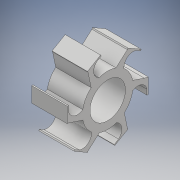
# Autodesk Inventor part: mtv_gear6_1-15
Saved by Autodesk Inventor 2018 (Build 220112000, 112)
## iProperties
Created: 2019-01-16
Part Number: mtv_gear6_1-15
Material: Generic
Document SubType Name: Modeling
Designer: aditya
Density: 1 g/cm^3
Appearance: Default
Author: aditya
Autodesk Inventor part; units mm, degrees
ref_plane "YZ Plane" through (0, 0, 0) normal (1, 0, 0) x (0, 1, 0)
ref_plane "XZ Plane" through (0, 0, 0) normal (0, 1, 0) x (-1, 0, 0)
ref_plane "XY Plane" through (0, 0, 0) normal (0, 0, 1) x (1, 0, 0)
sketch "Sketch1" plane through (0, 0, 0) normal (1, 0, 0) x (0, 1, 0)
  circle A0 centre (0, 0) radius 1.75
  circle A1 centre (0, 0) radius 2.5
  dimension "d0" = 3.5
  dimension "d1" = 5
  constraints: 2 centre point, 2 coincident
  measures "d0" diameter of A0
  measures "d1" diameter of A1
extrude "Extrusion1" add sketch "Sketch1" along normal blind 3.5
sketch "Sketch2" plane through (3.5, 0, 0) normal (1, 0, 0) x (0, 0, -1)
  circle A0 centre (0, 0) radius 2.5 construction
  line L0 (0, 2.5) -> (0, 2.375) construction
  line L1 (0, 2.375) -> (0.25, 2.375) construction
  line L2 (0.25, 2.375) -> (-0.25, 2.375) construction
  line L3 (-0.25, 2.375) -> (0.25, 2.375)
  line L4 (0, 2.375) -> (-0.5, 2.375)
  line L5 (-0.5, 2.375) -> (0.5, 2.375)
  line L6 (0, 2.375) -> (0, 3.875) construction
  line L7 (0, 3.875) -> (1, 3.875) construction
  line L8 (0, 3.875) -> (1, 3.875)
  line L9 (0, 3.875) -> (-0.5, 2.375)
  arc A1 (1, 3.875) -> (0.5, 2.375) centre (1.158, 2.989) ccw
  line L10 (0, 3.875) -> (1.5, 3.875)
  line L11 (1.5, 3.875) -> (1.5, 4)
  line L12 (1.5, 4) -> (0, 4)
  line L13 (0, 4) -> (0, 3.875)
  dimension "d4" = 0.125
  dimension "d5" = 0.25
  dimension "d6" = 0.5
  dimension "d11" = 0.5
  dimension "d12" = 1
  dimension "d14" = 1
  dimension "d15" = 0.9
  dimension "d16" = 1.5
  dimension "d17" = 0.125
  constraints: 28 end point, 3 equal length, 3 perpendicular, 3 point on line, 2 horizontal, 2 point on circle, 1 centre point, 1 vertical, 1 vertical alignment, 1 other
  measures "d4" distance of L0.start L0.end
  measures "d5" distance of L0.end L1.end
  measures "d6" distance of L1.end L2.end
  measures "d11" distance of L0.end L4.end
  measures "d12" distance of L4.end L5.end
  measures "d14" distance of L6.end L7.end
  measures "d15" radius of A1
  measures "d16" distance of L12.end L11.end
  measures "d17" distance of L11.end L10.end
extrude "Extrusion2" add sketch "Sketch2" against normal blind 3.5
fillet "Fillet1" radius 2 1 edges at (1.75, 3.875, 0)
pattern_circular "Circular Pattern1" count 6 over 360 about axis through (0, 0, 0) along (1, 0, 0) of "Extrusion2"
body "Solid1"
